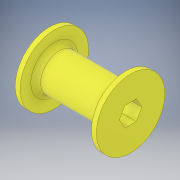
# Autodesk Inventor part: CLB_061_Winch
Saved by Autodesk Inventor 2018.3 (Build 223284000, 284)
## iProperties
Created: 2020-02-17
Part Number: CLB_061_Winch
Material: ABS Plastic
Document SubType Name: Modeling
Designer: user
Mass: 32.3011 g
Surface Area: 158.42 cm^2
Volume: 30.4727 cm^3
Density: 1.06 g/cm^3
Appearance: Smooth - Yellow
Author: user
Autodesk Inventor part; units mm, degrees
ref_plane "YZ Plane" through (0, 0, 0) normal (1, 0, 0) x (0, 1, 0)
ref_plane "XZ Plane" through (0, 0, 0) normal (0, 1, 0) x (-1, 0, 0)
ref_plane "XY Plane" through (0, 0, 0) normal (0, 0, 1) x (1, 0, 0)
sketch "Sketch1" plane through (0, 0, 0) normal (0, 0, 1) x (1, 0, 0)
  line L0 (0, 0) -> (3.175, 0)
  line L1 (3.175, 15.24) -> (3.175, 22.225)
  line L2 (3.175, 22.225) -> (0, 22.225)
  line L3 (0, 22.225) -> (0, 0)
  line L4 (0, 0) -> (52.705, 0)
  line L5 (52.705, 0) -> (52.705, 12.065)
  line L6 (46.355, 12.065) -> (6.35, 12.065)
  line L7 (0, 12.065) -> (0, 0)
  line L8 (52.705, 0) -> (49.53, 0)
  line L9 (49.53, 15.24) -> (49.53, 22.225)
  line L10 (49.53, 22.225) -> (52.705, 22.225)
  line L11 (52.705, 22.225) -> (52.705, 0)
  arc A0 (3.175, 15.24) -> (6.35, 12.065) centre (6.35, 15.24) ccw
  arc A1 (46.355, 12.065) -> (49.53, 15.24) centre (46.355, 15.24) ccw
  dimension "d0" = 52.705
  dimension "d1" = 22.225
  dimension "d2" = 12.065
  dimension "d3" = 3.175
  dimension "d4" = 3.175
  dimension "d5" = 3.175
  constraints: 24 end point, 6 parallel, 4 point on circle, 4 point on line, 4 tangent, 3 horizontal, 3 perpendicular, 2 centre point, 2 equal length
  measures "d0" distance of L0.start L4.end
  measures "d1" distance of L2.end L0.start
  measures "d2" distance between parallel lines of L0 L6
  measures "d3" distance of L1.end L2.end
  measures "d4" radius of A0
  measures "d5" radius of A1
revolve "Revolution1" add sketch "Sketch1" angle 360 about axis through (0, 0, 0) along (1, 0, 0)
sketch "Sketch2" plane through (52.705, 0, 0) normal (1, 0, 0) x (0, 0, -1)
  line L0 (7.3323, 0) -> (3.6662, -6.35)
  line L1 (3.6662, -6.35) -> (-3.6662, -6.35)
  line L2 (-3.6662, -6.35) -> (-7.3323, 0)
  line L3 (-7.3323, 0) -> (-3.6662, 6.35)
  line L4 (-3.6662, 6.35) -> (3.6662, 6.35)
  line L5 (3.6662, 6.35) -> (7.3323, 0)
  point P0 (0, 0)
  point P1 (0, 0)
  dimension "d7" = 12.7
  constraints: 12 end point, 1 coincident, 1 horizontal, 13 other
  measures "d7" distance between parallel lines of L1 L4
extrude "Extrusion1" cut sketch "Sketch2" against normal through all
body "Solid1"
